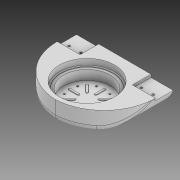
# Autodesk Inventor part: J1_NewBaseHDSide
Saved by Autodesk Inventor 2020 (Build 240168000, 168)
## iProperties
Created: 2021-06-11
Part Number: J1_NewBaseHDSide
Material: Generic
Document SubType Name: Modeling
Designer: DDeGo
Density: 1 g/cm^3
Appearance: Default
Author: DDeGo
Autodesk Inventor part; units mm, degrees
ref_plane "YZ Plane" through (0, 0, 0) normal (1, 0, 0) x (0, 1, 0)
ref_plane "XZ Plane" through (0, 0, 0) normal (0, 1, 0) x (-1, 0, 0)
ref_plane "XY Plane" through (0, 0, 0) normal (0, 0, 1) x (1, 0, 0)
sketch "Sketch1" plane through (0, 0, 0) normal (0, 0, 1) x (1, 0, 0)
  line L0 (-45, -85) -> (45, -85)
  line L1 (85, -45) -> (85, 45)
  line L2 (45, 85) -> (-45, 85)
  line L3 (-85, 45) -> (-85, -45)
  line L4 (-85, -85) -> (85, 85) construction
  line L5 (85, -85) -> (-85, 85) construction
  arc A0 (-45, 85) -> (-85, 45) centre (-45, 45) ccw
  arc A1 (85, 45) -> (45, 85) centre (45, 45) ccw
  arc A2 (45, -85) -> (85, -45) centre (45, -45) ccw
  arc A3 (-85, -45) -> (-45, -85) centre (-45, -45) ccw
  line L6 (-45, 52) -> (45, 52)
  arc A4 (52, 45) -> (45, 52) centre (45, 45) ccw
  line L7 (52, 45) -> (52, -45)
  arc A5 (45, -52) -> (52, -45) centre (45, -45) ccw
  line L8 (45, -52) -> (-45, -52)
  arc A6 (-52, -45) -> (-45, -52) centre (-45, -45) ccw
  line L9 (-52, -45) -> (-52, 45)
  arc A7 (-45, 52) -> (-52, 45) centre (-45, 45) ccw
  point P0 (0, 0)
  dimension "d0" = 170
  dimension "d1" = 170
  dimension "d2" = 40
  dimension "d3" = 33
  dimension "d36" = 104
  constraints: 20 end point, 16 point on circle, 8 centre point, 8 point on line, 8 tangent, 4 parallel, 3 equal radius, 2 midpoint, 2 perpendicular, 1 horizontal, 7 other
  measures "d0" distance between parallel lines of L1 L3
  measures "d1" distance between parallel lines of L2 L0
  measures "d2" radius of A0
  measures "d3" distance between parallel lines of L3 L9
  measures "d36" distance between parallel lines of L7 L9
extrude "Extrusion1" add sketch "Sketch1" along normal blind 120
sketch "Sketch2" plane through (85, -45, 0) normal (1, 0, 0) x (0, 0, -1)
  line L0 (0, -7) -> (-120, -7) construction
  line L1 (0, -7) -> (-120, -7) construction
  line L2 (0, 97) -> (-120, 97) construction
  line L3 (0, 97) -> (-120, 97) construction
  line L4 (0, 0) -> (0, 90) construction
  line L5 (-120, -7) -> (-120, 97)
  line L6 (-120, 130) -> (-120, 90) construction
  line L7 (-120, 0) -> (-120, 90) projected
  line L8 (-120, -7) -> (-32, -7)
  line L9 (-12, 13) -> (-12, 77)
  line L10 (-32, 97) -> (-120, 97)
  arc A0 (-32, -7) -> (-12, 13) centre (-32, 13) ccw
  arc A1 (-12, 77) -> (-32, 97) centre (-32, 77) ccw
  point P0 (0, 45)
  dimension "d7" = 12
  dimension "d8" = 20
  constraints: 8 end point, 4 point on circle, 4 tangent, 3 collinear, 2 centre point, 2 point on line, 1 equal radius, 1 perpendicular
  measures "d7" distance between parallel lines of L4 L9
  measures "d8" radius of A0
extrude "Extrusion2" cut sketch "Sketch2" against normal through all
sketch "Sketch3" plane through (-45, 85, 0) normal (0, 1, 0) x (1, 0, 0)
  line L0 (0, -120) -> (90, -120) construction
  line L1 (129.3827, -32) -> (90, -32) construction
  line L2 (90, 0) -> (90, -120) construction
  line L3 (90, -120) -> (0, -120) construction
  arc A0 (41.3827, -120) -> (129.3827, -32) centre (41.3827, -32) ccw
  line L4 (129.3827, -32) -> (129.3827, -120)
  line L5 (129.3827, -120) -> (41.3827, -120)
  line L6 (45, 0) -> (45, -120) construction
  arc A1 (-39.3827, -32) -> (48.6173, -120) centre (48.6173, -32) ccw
  line L7 (-39.3827, -32) -> (-39.3827, -120)
  line L8 (-39.3827, -120) -> (48.6173, -120)
  point P0 (0, -32)
  constraints: 10 end point, 5 symmetric about line, 4 point on circle, 3 tangent, 2 centre point, 1 line through centre, 1 midpoint, 1 perpendicular, 1 point on line, 1 vertical, 1 other
extrude "Extrusion3" cut sketch "Sketch3" against normal through all
sketch "Sketch4" plane through (0, 0, 0) normal (1, 0, 0) x (0, 1, 0)
  line L0 (-52, 119.9256) -> (-52, 32) construction
  line L1 (-52, 0) -> (-52, 32) construction
  line L2 (-52, 0) -> (-52, 32) construction
  line L3 (-52, 32) -> (-52, 119.9256) construction
  line L4 (-52, 65) -> (-79.6, 65)
  line L5 (-79.6, 65) -> (-79.6, 105.075)
  line L6 (-79.6, 105.075) -> (-63.1, 105.075)
  line L7 (-63.1, 105.075) -> (-63.1, 109.55)
  line L8 (-63.1, 109.55) -> (-62.1, 109.55)
  line L9 (-62.1, 109.55) -> (-62.1, 112.55)
  line L10 (-62.1, 112.55) -> (-52, 112.55)
  line L11 (-52, 112.55) -> (-52, 65)
  line L12 (-52, 65) -> (52, 65) construction
  line L13 (52, 120) -> (52, 32) construction
  line L14 (52, 65) -> (52, 76.05)
  line L15 (52, 65) -> (83, 65)
  line L16 (83, 65) -> (83, 74.55)
  line L17 (83, 74.55) -> (82.4, 74.55)
  line L18 (82.4, 74.55) -> (82.4, 76.05)
  line L19 (82.4, 76.05) -> (75.4, 76.05)
  line L20 (75.4, 76.05) -> (75.4, 100)
  line L21 (75.4, 100) -> (60.5, 100)
  line L22 (60.5, 100) -> (60.5, 74.55)
  line L23 (60.5, 74.55) -> (59, 74.55)
  line L24 (59, 74.55) -> (59, 76.05)
  line L25 (59, 76.05) -> (52, 76.05)
  line L26 (85, 0) -> (85, 105.3509) projected
  point P0 (0, 0)
  point P1 (52, 119.9256)
  dimension "d13" = 47.55
  dimension "d14" = 10.1
  dimension "d15" = 3
  dimension "d16" = 1
  dimension "d17" = 40.075
  dimension "d18" = 17.5
  dimension "d19" = 65
  dimension "d21" = 11.05
  dimension "d22" = 0.6
  dimension "d23" = 1.5
  dimension "d25" = 7
  dimension "d26" = 1.5
  dimension "d27" = 1.5
  dimension "d29" = 35
  dimension "d30" = 2
  dimension "d31" = 14.9
  constraints: 42 end point, 14 perpendicular, 4 point on line, 3 collinear, 3 horizontal, 1 parallel, 1 vertical
  measures "d13" distance between parallel lines of L4 L10
  measures "d14" distance of L9.end L10.end
  measures "d15" distance of L8.end L9.end
  measures "d16" distance of L7.end L8.end
  measures "d17" distance between parallel lines of L4 L6
  measures "d18" distance between parallel lines of L9 L5
  measures "d19" distance from line of L4 L2.start
  measures "d21" distance between parallel lines of L15 L25
  measures "d22" distance of L16.end L17.end
  measures "d23" distance of L17.end L18.end
  measures "d25" distance of L24.end L14.end
  measures "d26" distance of L22.end L23.end
  measures "d27" distance of L23.end L24.end
  measures "d29" distance between parallel lines of L15 L21
  measures "d30" distance between parallel lines of L26 L16
  measures "d31" distance between parallel lines of L22 L20
revolve "Revolution1" cut sketch "Sketch4" angle 360 about axis through (0, -52, 65) along (0, -1, 0)
sketch "Sketch5" plane through (0, 75.4, 65) normal (0, -1, 0) x (1, 0, 0)
  line L0 (-45, -65) -> (45, -65) construction
  line L1 (-20, -65) -> (-33.9793, -8.391)
  circle A0 centre (0, 0) radius 35 projected
  line L2 (33.0124, 11.6268) -> (60, -65)
  line L3 (60, -65) -> (-20, -65)
  point P0 (0, -65)
  dimension "d32" = 60
  dimension "d33" = 20
  constraints: 6 end point, 2 point on circle, 2 tangent, 1 horizontal, 1 point on line
  measures "d32" distance of L2.end point (0, -65)
  measures "d33" distance of L1.start point (0, -65)
extrude "Extrusion4" cut sketch "Sketch5" along normal up to surface (14.9 mm away) contours L1 A0 L2 L3
sketch "Sketch6" plane through (0, 0, 0) normal (0, 0, -1) x (-1, 0, 0)
  line L0 (-60, 60.5) -> (-60, 75.4) construction
  line L1 (-60, 75.4) -> (20, 75.4) construction
  line L2 (20, 75.4) -> (20, 60.5) construction
  line L3 (20, 60.5) -> (-60, 60.5) construction
  line L4 (85, 45) -> (85, -45) construction
  arc A0 (85, 45) -> (45, 85) centre (45, 45) ccw construction
  line L5 (-45, 85) -> (45, 85) construction
  arc A1 (-45, 85) -> (-85, 45) centre (-45, 45) ccw construction
  line L6 (-85, -45) -> (-85, 45) construction
  arc A2 (-85, -45) -> (-45, -85) centre (-45, -45) ccw construction
  line L7 (45, -85) -> (-45, -85) construction
  arc A3 (45, -85) -> (85, -45) centre (45, -45) ccw construction
  line L8 (-52, 45) -> (-52, -45) construction
  arc A4 (-45, 52) -> (-52, 45) centre (-45, 45) ccw construction
  line L9 (45, 52) -> (-45, 52) construction
  arc A5 (52, 45) -> (45, 52) centre (45, 45) ccw construction
  line L10 (52, -45) -> (52, 45) construction
  arc A6 (45, -52) -> (52, -45) centre (45, -45) ccw construction
  line L11 (-45, -52) -> (45, -52) construction
  arc A7 (-52, -45) -> (-45, -52) centre (-45, -45) ccw construction
  arc A8 (75.5, 45) -> (45, 75.5) centre (45, 45) ccw construction
  line L12 (75.5, 45) -> (75.5, -45) construction
  arc A9 (45, -75.5) -> (75.5, -45) centre (45, -45) ccw construction
  line L13 (45, -75.5) -> (-45, -75.5) construction
  arc A10 (-75.5, -45) -> (-45, -75.5) centre (-45, -45) ccw construction
  line L14 (-75.5, -45) -> (-75.5, 45) construction
  arc A11 (-45, 75.5) -> (-75.5, 45) centre (-45, 45) ccw construction
  line L15 (-45, 75.5) -> (45, 75.5) construction
  line L16 (45, 45) -> (45, 75.5) construction
  line L17 (45, 45) -> (0, 0) construction
  line L18 (45, 45) -> (75.5, 45) construction
  circle A12 centre (45, 75.5) radius 3.2
  circle A13 centre (75.5, 45) radius 3.2
  circle A14 centre (-75.5, 45) radius 3.2
  circle A15 centre (-45, 75.5) radius 3.2
  circle A16 centre (-45, -75.5) radius 3.2
  circle A17 centre (-75.5, -45) radius 3.2
  circle A18 centre (75.5, -45) radius 3.2
  circle A19 centre (45, -75.5) radius 3.2
  dimension "d37" = 9.5
  dimension "d38" = 45
  dimension "d39" = 6.4
  dimension "d42" = 360
  constraints: 14 end point, 12 centre point, 8 point on circle, 2 coincident, 2 point on line, 1 equal radius, 25 other
  measures "d37" distance between parallel lines of L4 L12
  measures "d38" angle of L17 L16
  measures "d39" diameter of A13
extrude "Extrusion5" cut sketch "Sketch6" against normal blind 12.5
fillet "Fillet1" radius 10 10 edges at (-52, 38.9292, 13.2387) (-52, 0, 12) (-52, -38.9292, 13.2387) (-49.3951, -50.4482, 24.2758) (-49.3957, 50.4477, 24.2746) (49.3951, 50.4482, 24.2758) (52, 0, 12) (52, -38.9292, 13.2387) (49.3957, -50.4477, 24.2746) (52, 38.9292, 13.2387)
sketch "Sketch9" plane through (-45, -52, 0) normal (0, 1, 0) x (1, 0, 0)
  line L0 (90, -23.579) -> (129.6683, -23.579) construction
  line L1 (90, 0) -> (90, -32) construction
  circle A0 centre (117.3827, -23.579) radius 1.9
  circle A1 centre (97, -23.579) radius 1.9
  point P0 (45, 0)
  dimension "d51" = 3.8
  dimension "d52" = 12
  dimension "d53" = 7
  constraints: 3 point on line, 2 centre point, 2 end point, 1 equal radius, 1 horizontal, 2 other
  measures "d51" diameter of A0
  measures "d52" horizontal distance of A0.centre point (129.383, -32)
  measures "d53" distance from line of L1 A1.centre
extrude "Extrusion8" cut sketch "Sketch9" along normal blind 5 and the other way blind 17
mirror "Mirror1" about plane through (0, 0, 0) normal (1, 0, 0) of "Extrusion8"
sketch "Sketch7" plane through (-45, -52, 0) normal (0, 1, 0) x (1, 0, 0)
  line L0 (129.3827, -32) -> (90, -32) projected
  line L1 (90, -32) -> (140.9289, -32)
  line L2 (140.9289, -32) -> (140.9289, 10.3254)
  line L3 (140.9289, 10.3254) -> (90, 10.3254)
  line L4 (90, 10.3254) -> (90, -32)
  line L5 (0, 0) -> (0, -32) projected
  line L6 (0, -32) -> (-66.1157, -32)
  line L7 (-66.1157, -32) -> (-66.1157, 14.7218)
  line L8 (-66.1157, 14.7218) -> (0, 14.7218)
  line L9 (0, 14.7218) -> (0, -32)
  point P0 (45, 0)
  constraints: 16 end point, 4 parallel, 2 horizontal, 2 perpendicular
extrude "Extrusion6" cut sketch "Sketch7" against normal blind 5
sketch "Sketch8" plane through (-45, -52, 0) normal (0, 1, 0) x (1, 0, 0)
  circle A0 centre (45, -42.7185) radius 303.5157
  point P0 (45, 0)
  constraints: 1 centre point
extrude "Extrusion7" cut sketch "Sketch8" along normal through all
sketch "Sketch10" plane through (0, -79.6, 65) normal (0, 1, 0) x (1, 0, 0)
  line L0 (0, 0) -> (0, 22.5) construction
  line L1 (0, 30) -> (0, 15) construction
  line L2 (-2, 30) -> (-2, 15)
  line L3 (2, 15) -> (2, 30)
  arc A0 (2, 30) -> (-2, 30) centre (0, 30) ccw
  arc A1 (-2, 15) -> (2, 15) centre (0, 15) ccw
  circle A2 centre (0, 0) radius 40.075 construction
  point P0 (0, 65)
  dimension "d58" = 15
  dimension "d59" = 2
  dimension "d60" = 22.5
  constraints: 10 end point, 4 point on circle, 4 tangent, 2 centre point, 1 coincident, 1 midpoint, 1 parallel, 1 point on line, 1 vertical
  measures "d58" distance of L1.start L1.end
  measures "d59" radius of A0
  measures "d60" distance of L0.start L0.end
extrude "Extrusion9" add sketch "Sketch10" along normal blind 0.8
fillet "Fillet3" radius 10 4 edges at (-23.4976, -85, 115.7185) (-75.5189, -70.8573, 70.4899) (23.4976, -85, 115.7185) (75.456, -70.9313, 70.6189)
fillet "Fillet4" radius 0.5 4 edges at (0, -78.8, 52) (2, -78.8, 42.5) (0, -78.8, 33) (-2, -78.8, 42.5)
sketch "Sketch11" plane through (0, -79.6, 65) normal (0, 1, 0) x (1, 0, 0)
  circle A0 centre (0, 0) radius 40.075 construction
  line L0 (0, 0) -> (-11.4805, 27.7164) construction
  line L1 (0, 0) -> (0, -9.8921) construction
  circle A1 centre (-11.4805, 27.7164) radius 1.75
  point P0 (0, 65)
  dimension "d70" = 30
  dimension "d71" = 3.5
  dimension "d75" = 22.5
  constraints: 4 end point, 1 centre point, 1 coincident, 1 vertical
  measures "d70" distance of L0.start L0.end
  measures "d71" diameter of A1
  measures "d75" angle of L1 L0
extrude "Extrusion10" cut sketch "Sketch11" against normal through all
ref_plane "Work Plane1" through (0, -81.6, 65) normal (0, 1, 0) x (1, 0, 0)
sketch "Sketch12" plane through (0, -81.6, 65) normal (0, 1, 0) x (1, 0, 0)
  circle A0 centre (-11.4805, 27.7164) radius 1.75 construction
  circle A1 centre (-11.4805, 27.7164) radius 3
  point P0 (0, 65)
  dimension "d77" = 6
  constraints: 1 centre point, 1 coincident
  measures "d77" diameter of A1
extrude "Extrusion11" cut sketch "Sketch12" against normal through all
pattern_circular "Circular Pattern1" count 8 over 360 about axis through (0, -71.35, 65) along (0, 1, 0) of "Extrusion11", "Extrusion10", "Fillet4", "Extrusion9"
sketch "Sketch13" plane through (-45, -85, 0) normal (0, -1, 0) x (1, 0, 0)
  circle A0 centre (45, 65) radius 40.075 construction
  circle A1 centre (45, 65) radius 26
  circle A2 centre (45, 65) radius 34
  circle A3 centre (72.7164, 76.4805) radius 3 construction
  circle A4 centre (17.2836, 76.4805) radius 1.75 construction
  circle A5 centre (17.2836, 76.4805) radius 4
  circle A6 centre (72.7164, 76.4805) radius 4
  circle A7 centre (33.5195, 92.7164) radius 3 construction
  circle A8 centre (33.5195, 92.7164) radius 4
  circle A9 centre (56.4805, 92.7164) radius 1.75 construction
  circle A10 centre (56.4805, 92.7164) radius 4
  point P0 (45, 0)
  point P1 (69.0209, 74.9498)
  point P2 (54.9498, 89.0209)
  point P3 (58.0112, 96.4119)
  point P4 (76.4119, 78.0112)
  dimension "d83" = 1
  dimension "d84" = 1
  constraints: 6 centre point, 6 coincident, 4 tangent
extrude "Extrusion12" cut sketch "Sketch13" against normal blind 0.5 contours A1 A6 A2 A5 | A6 | A5 A2 A8 A1 | A5 | A1 A8 A2 A10 | A10 | A8
sketch "Sketch14" plane through (0, 0, 0) normal (0, 0, -1) x (-1, 0, 0)
  circle A0 centre (-45, -75.5) radius 3.2 projected
  circle A1 centre (45, -75.5) radius 3.2 projected
  line L0 (-45, -75.5) -> (45, -75.5) construction
  line L1 (0, -75.5) -> (0, -60.5) construction
  circle A2 centre (0, -60.5) radius 1.9
  circle A3 centre (30, -75.5) radius 1.9
  circle A4 centre (-30, -75.5) radius 1.9
  point P0 (0, 0)
  dimension "d87" = 15
  dimension "d88" = 15
  dimension "d89" = 15
  dimension "d90" = 3.8
  constraints: 4 end point, 3 centre point, 2 equal radius, 2 point on line, 1 coincident, 1 horizontal, 1 midpoint, 1 vertical
  measures "d87" distance of L1.start L1.end
  measures "d88" distance of L0.start A4.centre
  measures "d89" distance of L0.end A3.centre
  measures "d90" diameter of A2
extrude "Extrusion13" cut sketch "Sketch14" against normal blind 10 contours A2 | A3 | A4
body "Solid1"
